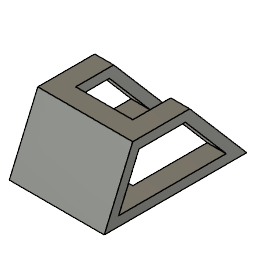
ex24aug29 (Autodesk Fusion 360 design; units mm, degrees)
part number: 2026-08-29-12-15-56-500
Autodesk Fusion 360 part; units mm, degrees
sketch "Sketch2" plane through (0, 0, 0) normal (1, 0, 0) x (0, 0, -1)
  line L0 (0, 0) -> (30, 70)
  line L1 (30, 70) -> (90, 70)
  line L2 (90, 70) -> (150, 0)
  line L3 (150, 0) -> (0, 0)
  line L4 (36.594, 60) -> (85.4007, 60)
  line L5 (85.4007, 60) -> (128.2578, 10)
  line L6 (128.2578, 10) -> (15.1654, 10)
  line L7 (15.1654, 10) -> (36.594, 60)
  dimension "d9" = 10
  dimension "d10" = 70
  dimension "d11" = 30
  dimension "d12" = 60
  dimension "d13" = 60
  constraint coincident L0.start L3.end
  constraint horizontal L1
  constraint parallel L1 L3
  measures "d10" vertical distance of L0.start L0.end
  measures "d11" horizontal distance of L0.start L0.end
  measures "d12" distance of L0.end L1.end
  measures "d13" horizontal distance of L1.end L2.end
extrude "Extrude1" add sketch "Sketch2" along normal blind 100
sketch "Sketch3" plane through (0, 70, 0) normal (0, 1, 0) x (-1, 0, 0)
  line L0 (0, -90) -> (0, -30)
  line L1 (0, -30) -> (-100, -30)
  line L2 (-100, -30) -> (-100, -90)
  line L3 (-100, -90) -> (0, -90)
  line L4 (-100, -30) -> (0, -30) construction
  line L5 (-50, -30) -> (-50, -100) construction
  line L6 (-20, -150) -> (-80, -150)
  line L7 (-80, -150) -> (-80, -50)
  line L8 (-80, -50) -> (-20, -50)
  line L9 (-20, -50) -> (-20, -150)
  line L10 (-20, -150) -> (-80, -50) construction
  line L11 (-80, -150) -> (-20, -50) construction
  point P0 (-50, -100)
  dimension "d19" = 70
  dimension "d20" = 60
  dimension "d21" = 100
  constraint coincident L1.end L2.start
  constraint coincident L0.end L1.start
  constraint midpoint L4 L5.start
  constraint perpendicular L4 L5
  constraint horizontal L6
  constraint perpendicular L6 L7
  constraint parallel L6 L8
  constraint parallel L7 L9
  constraint coincident L10 P0
  constraint coincident L11 P0
  constraint coincident P0 L5.end
  measures "d19" distance of L5.start P0
  measures "d20" distance of L7.end L8.end
  measures "d21" distance of L6.end L7.end
extrude "Extrude2" cut sketch "Sketch3" against normal through all contours L3 L6 L7 L9 | L3 L7 L8 L9
